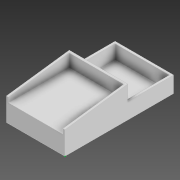
# Autodesk Inventor part: PB en arduino
Saved by Autodesk Inventor 2020.2 (Build 242310000, 310)
## iProperties
Created: 2019-12-09
Part Number: PB en arduino
Material: Generic
Document SubType Name: Modeling
Designer: Berkant
Density: 1 g/cm^3
Appearance: Default
Author: Berkant
Autodesk Inventor part; units mm, degrees
ref_plane "YZ Plane" through (0, 0, 0) normal (1, 0, 0) x (0, 1, 0)
ref_plane "XZ Plane" through (0, 0, 0) normal (0, 1, 0) x (-1, 0, 0)
ref_plane "XY Plane" through (0, 0, 0) normal (0, 0, 1) x (1, 0, 0)
sketch "Sketch1" plane through (0, 0, 0) normal (0, 1, 0) x (-1, 0, 0)
  line L0 (0, 0) -> (84, 0)
  line L1 (84, 0) -> (84, -156)
  line L2 (84, -156) -> (0, -156)
  line L3 (0, -156) -> (0, 0)
  line L4 (84, 0) -> (81, 0)
  line L5 (81, 0) -> (81, -3) construction
  line L6 (81, -3) -> (84, -3) construction
  line L7 (84, -3) -> (84, 0)
  line L8 (0, -156) -> (3, -156)
  line L9 (3, -156) -> (3, -153) construction
  line L10 (3, -153) -> (0, -153) construction
  line L11 (0, -153) -> (0, -156)
  line L12 (81, -3) -> (0, -3) construction
  dimension "d0" = 84
  dimension "d1" = 156
  constraints: 26 end point, 6 parallel, 4 perpendicular, 3 horizontal, 1 point on line
  measures "d0" distance of L1.end L2.end
  measures "d1" distance of L0.end L1.end
extrude "Extrusion1" add sketch "Sketch1" along normal blind 3
sketch "Sketch2" plane through (0, 3, 0) normal (0, 1, 0) x (1, 0, 0)
  line L0 (-84, 0) -> (0, 0) projected
  line L1 (-84, 0) -> (-42, 0)
  line L2 (-81, 3) -> (-3, 3)
  line L3 (-3, 3) -> (-3, 153)
  line L4 (-3, 153) -> (-81, 153)
  line L5 (-81, 153) -> (-81, 3)
  line L6 (-42, 0) -> (-42, 3)
  line L7 (-81, 3) -> (-47.5, 3)
  line L8 (0, 0) -> (0, 156) projected
  line L9 (-84, 0) -> (0, 0)
  line L10 (0, 0) -> (0, 156)
  line L11 (0, 156) -> (-84, 156)
  line L12 (-84, 156) -> (-84, 0)
  line L13 (-84, 156) -> (-84, 0) projected
  dimension "d12" = 42
  dimension "d13" = 78
  dimension "d14" = 150
  dimension "d15" = 3
  dimension "d16" = 33.5
  constraints: 22 end point, 4 parallel, 2 horizontal, 2 midpoint, 2 perpendicular, 1 point on line, 1 vertical
  measures "d12" distance of L0.start L1.end
  measures "d13" distance of L4.end L3.end
  measures "d14" distance of L3.end L2.end
  measures "d15" distance of L6.end L1.end
  measures "d16" distance of L2.start L7.end
extrude "Extrusion2" add sketch "Sketch2" along normal blind 20
sketch "Sketch3" plane through (0, 0, 0) normal (1, 0, 0) x (0, 0, -1)
  line L0 (156, 23) -> (0, 23) projected
  line L1 (0, 23) -> (90.225, 23)
  line L2 (90.225, 23) -> (90.225, 26)
  line L3 (90.225, 26) -> (0, 26)
  line L4 (0, 26) -> (0, 23)
  point P0 (0, 0)
  dimension "d19" = 90.225
  dimension "d20" = 3
  constraints: 8 end point, 2 parallel, 1 horizontal, 1 perpendicular
  measures "d19" distance of L3.end L2.end
  measures "d20" distance of L2.end L1.end
extrude "Extrusion3" add sketch "Sketch3" against normal up to surface (84 mm away)
sketch "Sketch4" plane through (0, 0, 0) normal (1, 0, 0) x (0, 0, -1)
  line L0 (0, 33) -> (90.225, 44.756)
  line L1 (0, 26) -> (0, 33)
  line L2 (90.225, 23) -> (90.225, 26) projected
  line L3 (0, 26) -> (90.225, 26)
  line L4 (90.225, 26) -> (90.225, 44.756)
  constraints: 8 end point, 1 horizontal, 1 perpendicular, 1 vertical
sketch "Sketch5" plane through (-84, 0, 0) normal (0, 0, 1) x (1, 0, 0)
  line L0 (3, 33) -> (3, 26)
  line L1 (3, 26) -> (81, 26)
  line L2 (81, 26) -> (81, 33)
  line L3 (81, 26) -> (3, 26)
  line L4 (3, 26) -> (3, 44.756)
  line L5 (3, 44.756) -> (81, 44.756)
  line L6 (81, 44.756) -> (81, 26)
  line L7 (3, 33) -> (81, 33)
  point P0 (84, 0)
  point P1 (84, 33)
  dimension "d27" = 3
  dimension "d28" = 78
  dimension "d29" = 7
  constraints: 16 end point, 3 parallel, 1 horizontal, 1 perpendicular
  measures "d27" distance of point (84, 33) L2.end
  measures "d28" distance of L1.end L0.end
  measures "d29" distance of L0.end L0.start
sketch "Sketch6" plane through (0, 0, 0) normal (1, 0, 0) x (0, 0, -1)
  point P0 (0, 0)
extrude "Extrusion7" add sketch "Sketch4" against normal up to surface (84 mm away)
extrude "Extrusion10" cut sketch "Sketch5" against normal blind 87.25
body "Solid1"
